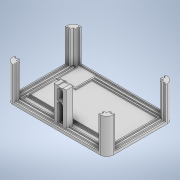
# Autodesk Inventor part: bottom
Saved by Autodesk Inventor 2021 (Build 250183000, 183)
## iProperties
Created: 2021-08-17
Part Number: bottom
Material: Generisch
Document SubType Name: Modeling
Designer: Tilman
Density: 1 g/cm^3
Appearance: Vorgabe
Author: Tilman
Autodesk Inventor part; units mm, degrees
ref_plane "YZ Plane" through (0, 0, 0) normal (1, 0, 0) x (0, 1, 0)
ref_plane "XZ Plane" through (0, 0, 0) normal (0, 1, 0) x (-1, 0, 0)
ref_plane "XY Plane" through (0, 0, 0) normal (0, 0, 1) x (1, 0, 0)
sketch "Skizze1" plane through (0, 0, 0) normal (0, 1, 0) x (-1, 0, 0)
  line L0 (0, 0) -> (-130, 0)
  line L1 (-140, -10) -> (-140, -90)
  line L2 (-130, -100) -> (0, -100)
  line L3 (10, -10) -> (10, -90)
  arc A0 (0, -100) -> (10, -90) centre (0, -90) ccw
  arc A1 (-140, -90) -> (-130, -100) centre (-130, -90) ccw
  arc A2 (-130, 0) -> (-140, -10) centre (-130, -10) ccw
  arc A3 (10, -10) -> (0, 0) centre (0, -10) ccw
  dimension "d0" = 150
  dimension "d1" = 100
  dimension "d2" = 10
  constraints: 8 end point, 8 point on circle, 7 tangent, 4 centre point, 3 equal radius, 2 horizontal, 2 parallel, 2 vertical
  measures "d0" distance between parallel lines of L1 L3
  measures "d1" distance between parallel lines of L0 L2
  measures "d2" radius of A2
extrude "Extrusion1" add sketch "Skizze1" along normal blind 2
sketch "Skizze2" plane through (0, 2, 0) normal (0, 1, 0) x (1, 0, 0)
  line L0 (0, 0) -> (130, 0) projected
  arc A0 (130, 0) -> (140, 10) centre (130, 10) ccw projected
  line L1 (140, 10) -> (140, 90) projected
  arc A1 (140, 90) -> (130, 100) centre (130, 90) ccw projected
  line L2 (130, 100) -> (0, 100) projected
  arc A2 (0, 100) -> (-10, 90) centre (0, 90) ccw projected
  line L3 (-10, 90) -> (-10, 10) projected
  arc A3 (-10, 10) -> (0, 0) centre (0, 10) ccw projected
  line L4 (0, 2) -> (130, 2)
  line L5 (130, 2) -> (130, 5.5)
  line L6 (130, 5.5) -> (0, 5.5)
  line L7 (0, 5.5) -> (0, 2)
  line L8 (138, 10) -> (134.5, 10)
  line L9 (134.5, 10) -> (134.5, 90)
  line L10 (134.5, 90) -> (138, 90)
  line L11 (138, 90) -> (138, 10)
  line L12 (130, 98) -> (0, 98)
  line L13 (0, 98) -> (0, 94.5)
  line L14 (0, 94.5) -> (130, 94.5)
  line L15 (130, 94.5) -> (130, 98)
  line L16 (-8, 90) -> (-4.5, 90)
  line L17 (-4.5, 90) -> (-4.5, 10)
  line L18 (-4.5, 10) -> (-8, 10)
  line L19 (-8, 10) -> (-8, 90)
  line L20 (65, 2) -> (65, 0) construction
  line L21 (0, 0) -> (130, 0) construction
  line L22 (138, 50) -> (140, 50) construction
  line L23 (140, 10) -> (140, 90) construction
  line L24 (65, 98) -> (65, 100) construction
  line L25 (130, 100) -> (0, 100) construction
  line L26 (-8, 50) -> (-10, 50) construction
  line L27 (-10, 90) -> (-10, 10) construction
  line L28 (140, 88) -> (138, 88)
  line L29 (134.5, 88) -> (132.5, 88)
  line L30 (132.5, 88) -> (132.5, 92.5)
  line L31 (132.5, 92.5) -> (128, 92.5)
  line L32 (128, 92.5) -> (128, 94.5)
  line L33 (128, 98) -> (128, 100)
  line L34 (140, 12) -> (138, 12)
  line L35 (134.5, 12) -> (132.5, 12)
  line L36 (132.5, 12) -> (132.5, 7.5)
  line L37 (132.5, 7.5) -> (128, 7.5)
  line L38 (128, 7.5) -> (128, 5.5)
  line L39 (128, 2) -> (128, 0)
  line L40 (2, 0) -> (2, 2)
  line L41 (2, 5.5) -> (2, 7.5)
  line L42 (2, 7.5) -> (-2.5, 7.5)
  line L43 (-2.5, 7.5) -> (-2.5, 12)
  line L44 (-2.5, 12) -> (-4.5, 12)
  line L45 (-8, 12) -> (-10, 12)
  line L46 (-10, 88) -> (-8, 88)
  line L47 (-4.5, 88) -> (-2.5, 88)
  line L48 (-2.5, 88) -> (-2.5, 92.5)
  line L49 (-2.5, 92.5) -> (2, 92.5)
  line L50 (2, 92.5) -> (2, 94.5)
  line L51 (2, 98) -> (2, 100)
  line L52 (-2, 92) -> (132, 92)
  line L53 (132, 92) -> (132, 8)
  line L54 (132, 8) -> (-2, 8)
  line L55 (-2, 8) -> (-2, 92)
  line L56 (130, 90) -> (0, 90)
  line L57 (0, 90) -> (0, 10)
  line L58 (0, 10) -> (130, 10)
  line L59 (130, 10) -> (130, 90)
  line L60 (-2.5, 92.5) -> (0, 90) construction
  line L61 (132.5, 92.5) -> (130, 90) construction
  line L62 (132.5, 7.5) -> (130, 10) construction
  line L63 (-2.5, 7.5) -> (0, 10) construction
  line L64 (2, 88) -> (128, 88)
  line L65 (128, 88) -> (128, 12)
  line L66 (128, 12) -> (2, 12)
  line L67 (2, 12) -> (2, 88)
  point P0 (130, 3.75)
  point P1 (128, 0)
  dimension "d5" = 3.5
  dimension "d6" = 2
  dimension "d7" = 2
  dimension "d12" = 2
  dimension "d13" = 2
  dimension "d14" = 0.5
  dimension "d15" = 2
  constraints: 120 end point, 42 point on line, 21 perpendicular, 20 equal length, 15 parallel, 9 midpoint, 7 horizontal alignment, 7 vertical alignment, 6 horizontal, 3 vertical, 6 other
  measures "d5" distance of L12.end L13.end
  measures "d6" distance of L24.start L24.end
  measures "d7" distance of L49.end L50.end
  measures "d12" distance between parallel lines of L13 L50
  measures "d13" distance between parallel lines of L52 L56
  measures "d14" distance between parallel lines of L48 L55
  measures "d15" distance between parallel lines of L56 L64
extrude "Extrusion2" add sketch "Skizze2" along normal blind 2 contours L40 L4 L39 L0 | L3 L46 L19 L45 | L34 L11 L28 L1 | L41 L42 L43 L44 L17 L47 L48 L49 L50 L14 L32 L31 L30 L29 L9 L35 L36 L37 L38 L6 | L2 L33 L12 L51 | L59 L58 L57 L56
extrude "Extrusion3" add sketch "Skizze2" along normal blind 50 contours A3 L3 L45 L19 L18 L17 L44 L43 L42 L41 L6 L7 L4 L40 L0 | L39 L4 L5 L6 L38 L37 L36 L35 L9 L8 L11 L34 L1 A0 L0 | L3 A2 L2 L51 L12 L13 L14 L50 L49 L48 L47 L17 L16 L19 L46 | L28 L11 L10 L9 L29 L30 L31 L32 L14 L15 L12 L33 L2 A1 L1
sketch "Skizze3" plane through (0, 2, 0) normal (0, 1, 0) x (1, 0, 0)
  line L0 (2, 88) -> (2, 12) projected
  line L1 (2, 12) -> (128, 12) projected
  line L2 (128, 12) -> (128, 88) projected
  line L3 (128, 88) -> (2, 88) projected
  line L4 (-2, 92) -> (-2, 8) projected
  line L5 (-2, 8) -> (132, 8) projected
  line L6 (132, 8) -> (132, 92) projected
  line L7 (132, 92) -> (-2, 92) projected
  line L8 (0, 90) -> (130, 90) projected
  line L9 (130, 90) -> (130, 10) projected
  line L10 (130, 10) -> (0, 10) projected
  line L11 (0, 10) -> (0, 90) projected
  line L12 (3, 19.5) -> (127, 19.5)
  line L13 (127, 19.5) -> (127, 21.5)
  line L14 (127, 21.5) -> (3, 21.5)
  line L15 (3, 21.5) -> (3, 19.5)
  line L16 (2, 22.5) -> (128, 22.5)
  line L17 (2, 12) -> (2, 88) projected
  line L18 (2, 18.5) -> (128, 18.5)
  line L19 (128, 12) -> (128, 88) projected
  point P0 (0, 0)
  point P1 (65, 19.5)
  point P2 (65, 8)
  dimension "d20" = 2
  dimension "d21" = 11.5
  dimension "d22" = 1
  dimension "d23" = 1
  dimension "d26" = 1
  constraints: 12 end point, 4 point on line, 3 horizontal, 2 midpoint, 2 parallel, 1 perpendicular, 1 vertical alignment
  measures "d20" distance of L12.end L13.end
  measures "d21" distance between parallel lines of L5 L12
  measures "d22" distance between parallel lines of L15 L0
  measures "d23" distance between parallel lines of L14 L16
  measures "d26" distance between parallel lines of L18 L12
extrude "Extrusion4" add sketch "Skizze3" along normal up to surface (2 mm away) contours L16 L2 L18 L0
sketch "Skizze4" plane through (0, 2, 0) normal (0, 1, 0) x (1, 0, 0)
  line L0 (128, 94.5) -> (2, 94.5) projected
  line L1 (2, 22.5) -> (2, 88) projected
  line L2 (2, 94.5) -> (28, 94.5)
  line L3 (28, 94.5) -> (28, 65.5)
  line L4 (28, 65.5) -> (2, 65.5)
  line L5 (2, 65.5) -> (2, 94.5)
  line L6 (2, 63.5) -> (30, 63.5)
  line L7 (30, 63.5) -> (30, 94.5)
  circle A0 centre (16, 61.5) radius 2
  circle A1 centre (16, 61.5) radius 0.95
  point P0 (0, 0)
  point P1 (2, 65.5)
  point P2 (16, 63.5)
  dimension "d27" = 26
  dimension "d28" = 29
  dimension "d31" = 2
  dimension "d32" = 2
  dimension "d54" = 1.9
  dimension "d55" = 4
  constraints: 12 end point, 2 centre point, 2 horizontal, 2 parallel, 2 perpendicular, 2 point on line, 1 coincident, 1 midpoint, 1 tangent, 1 vertical alignment
  measures "d27" distance of L3.end L4.end
  measures "d28" distance of L2.end L3.end
  measures "d31" distance between parallel lines of L4 L6
  measures "d32" distance between parallel lines of L7 L3
  measures "d54" diameter of A1
  measures "d55" diameter of A0
extrude "Extrusion5" cut sketch "Skizze4" along normal through all contours L3 L4 L1 L5 L0
extrude "Extrusion6" add sketch "Skizze4" along normal blind 2 contours L7 L6 L1 L4 L3 L0
extrude "Extrusion9" add sketch "Skizze4" along normal blind 5 contours A0
sketch "Skizze5" plane through (0, 4, 0) normal (0, 1, 0) x (1, 0, 0)
  line L0 (2, 65.5) -> (2, 90) construction
  line L1 (2, 90) -> (0, 90) construction
  line L2 (0, 90) -> (0, 10) construction
  line L3 (0, 10) -> (130, 10) construction
  line L4 (130, 10) -> (130, 90) construction
  line L5 (130, 90) -> (30, 90) construction
  line L6 (30, 90) -> (30, 92) construction
  line L7 (30, 92) -> (132, 92) construction
  line L8 (132, 92) -> (132, 8) construction
  line L9 (132, 8) -> (-2, 8) construction
  line L10 (-2, 8) -> (-2, 92) construction
  line L11 (-2, 92) -> (2, 92) construction
  line L12 (2, 92.5) -> (-2.5, 92.5) construction
  line L13 (-2.5, 92.5) -> (-2.5, 88) construction
  line L14 (-2.5, 88) -> (-4.5, 88) construction
  line L15 (-4.5, 88) -> (-4.5, 12) construction
  line L16 (-4.5, 12) -> (-2.5, 12) projected
  line L17 (-2.5, 12) -> (-2.5, 7.5) projected
  line L18 (-2.5, 7.5) -> (2, 7.5) projected
  line L19 (2, 7.5) -> (2, 5.5) projected
  line L20 (2, 5.5) -> (128, 5.5) construction
  line L21 (128, 5.5) -> (128, 7.5) projected
  line L22 (128, 7.5) -> (132.5, 7.5) projected
  line L23 (132.5, 7.5) -> (132.5, 12) projected
  line L24 (132.5, 12) -> (134.5, 12) projected
  line L25 (134.5, 12) -> (134.5, 88) construction
  line L26 (134.5, 88) -> (132.5, 88) construction
  line L27 (132.5, 88) -> (132.5, 92.5) construction
  line L28 (132.5, 92.5) -> (128, 92.5) construction
  line L29 (128, 92.5) -> (128, 94.5) construction
  line L30 (128, 94.5) -> (28, 94.5) construction
  line L31 (28, 94.5) -> (28, 65.5) construction
  line L32 (28, 65.5) -> (2, 65.5) construction
  line L33 (3, 19.5) -> (127, 19.5) construction
  line L34 (3, 21.5) -> (3, 19.5) projected
  line L35 (127, 21.5) -> (3, 21.5) construction
  line L36 (127, 19.5) -> (127, 21.5) projected
  line L37 (128, 18.5) -> (128, 12) projected
  line L38 (128, 12) -> (2, 12) construction
  line L39 (2, 12) -> (2, 18.5) projected
  line L40 (128, 18.5) -> (2, 18.5) construction
  line L41 (2, 63.5) -> (16, 63.5) construction
  line L42 (30, 63.5) -> (30, 88) construction
  line L43 (30, 88) -> (128, 88) construction
  line L44 (128, 88) -> (128, 22.5) construction
  line L45 (2, 22.5) -> (128, 22.5) construction
  line L46 (2, 22.5) -> (2, 63.5) construction
  line L47 (56, 5.5) -> (61, 5.5)
  line L48 (61, 5.5) -> (61, 15.5)
  line L49 (61, 15.5) -> (56, 15.5)
  line L50 (56, 15.5) -> (56, 5.5)
  line L51 (69, 15.5) -> (74, 15.5)
  line L52 (74, 15.5) -> (74, 5.5)
  line L53 (74, 5.5) -> (69, 5.5)
  line L54 (69, 5.5) -> (69, 15.5)
  line L55 (61, 10.5) -> (69, 10.5) construction
  line L56 (2, 92) -> (2, 92.5) projected
  line L57 (16, 63.5) -> (30, 63.5) projected
  point P0 (0, 0)
  point P1 (65, 5.5)
  point P2 (65, 10.5)
  dimension "d41" = 10
  dimension "d42" = 8
  dimension "d43" = 5
  constraints: 18 end point, 4 midpoint, 4 parallel, 2 horizontal, 2 horizontal alignment, 2 perpendicular, 1 collinear, 1 point on line, 1 vertical alignment
  measures "d41" distance of L49.end L47.start
  measures "d42" distance of L55.start L55.end
  measures "d43" distance of L47.start L47.end
extrude "Extrusion7" add sketch "Skizze5" along normal blind 49 and the other way blind 2
sketch "Skizze6" plane through (0, 2, -5.5) normal (0, 0, 1) x (1, 0, 0)
  line L0 (2, 2) -> (56, 2) projected
  line L1 (2, 2) -> (2, 50) projected
  line L2 (0, 50) -> (2, 50) projected
  line L3 (0, 0) -> (0, 50) projected
  line L4 (130, 0) -> (0, 0) projected
  line L5 (130, 0) -> (130, 50) projected
  line L6 (128, 50) -> (130, 50) projected
  line L7 (128, 2) -> (128, 50) projected
  line L8 (74, 2) -> (128, 2) projected
  line L9 (74, 2) -> (74, 51) projected
  line L10 (69, 51) -> (74, 51) projected
  line L11 (69, 51) -> (69, 2) projected
  line L12 (61, 2) -> (69, 2) projected
  line L13 (61, 51) -> (61, 2) projected
  line L14 (56, 51) -> (61, 51) projected
  line L15 (56, 2) -> (56, 51) projected
  line L16 (69, 51) -> (69, 2) projected
  line L17 (61, 0) -> (61, 51) projected
  arc A0 (69, 27) -> (61, 27) centre (65, 27) ccw
  line L18 (61, 32) -> (69, 32)
  arc A1 (69, 45) -> (61, 45) centre (65, 45) ccw
  line L19 (61, 50) -> (69, 50)
  point P0 (0, -2)
  dimension "d48" = 5
  dimension "d49" = 5
  dimension "d50" = 1
  dimension "d51" = 13
  constraints: 8 point on line, 4 end point, 4 horizontal alignment, 4 point on circle, 2 centre point, 2 horizontal
  measures "d48" distance from line of A0.centre L18
  measures "d49" distance from line of A1.centre L19
  measures "d50" distance between parallel lines of L10 L19
  measures "d51" distance from line of A1.start L18
extrude "Extrusion8" add sketch "Skizze6" against normal up to surface (10 mm away) contours L19 L11 A1 L13 | L18 L11 A0 L13
equation "\"d23\" = d22"
equation "\"d26\" = d23"
